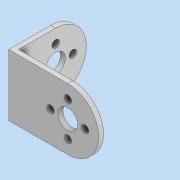
# Autodesk Inventor part: Bracket ANGULO
Saved by Autodesk Inventor 2021.4 (Build 254397000, 397)
## iProperties
Created: 2022-08-02
Part Number: Bracket ANGULO
Material: Generic
Document SubType Name: Modeling
Designer: ferbm
Density: 1 g/cm^3
Appearance: Default
Author: ferbm
Autodesk Inventor part; units mm, degrees
ref_plane "YZ Plane" through (0, 0, 0) normal (1, 0, 0) x (0, 1, 0)
ref_plane "XZ Plane" through (0, 0, 0) normal (0, 1, 0) x (-1, 0, 0)
ref_plane "XY Plane" through (0, 0, 0) normal (0, 0, 1) x (1, 0, 0)
sketch "Sketch1" plane through (0, 0, 0) normal (0, 0, 1) x (1, 0, 0)
  line L0 (0, 0) -> (24, 0)
  line L1 (24, 25) -> (0, 25)
  line L2 (0, 25) -> (0, 0)
  arc A0 (24, 0) -> (24, 25) centre (24, 12.5) ccw
  circle A1 centre (24, 12.5) radius 4
  circle A2 centre (24, 12.5) radius 7
  circle A3 centre (24, 19.5) radius 1.5
  circle A4 centre (17, 12.5) radius 1.5
  circle A5 centre (24, 5.5) radius 1.5
  circle A6 centre (31, 12.5) radius 1.5
  line L3 (24, 0) -> (24, 16.5)
  line L4 (24, 19.5) -> (24, 21)
  line L5 (0, 25) -> (2, 25)
  line L6 (2, 25) -> (2, 0)
  line L7 (2, 0) -> (0, 0)
  line L8 (0, 0) -> (0, 25)
  dimension "d2" = 8
  dimension "d3" = 14
  dimension "d4" = 3
  dimension "d0" = 24
  dimension "d1" = 25
  dimension "d7" = 360
  dimension "d11" = 2
  constraints: 18 end point, 5 parallel, 4 centre point, 3 perpendicular, 3 vertical alignment, 2 coincident, 2 horizontal, 2 point on circle, 2 tangent, 1 point on line, 15 other
  measures "d0" distance of L1.start L1.end
  measures "d1" distance of L0.end L1.start
  measures "d11" distance between parallel lines of L2 L6
extrude "Extrusion1" add sketch "Sketch1" along normal blind 2 contours L2 L1 L6 L0 | L6 L1 A0 L0 | A2 A4 A3 A6 A5
extrude "Extrusion2" add sketch "Sketch1" against normal blind 1 contours L2 L1 L6 L0
sketch "Sketch2" plane through (2, 0, 0) normal (1, 0, 0) x (0, 0, -1)
  line L0 (0, 25) -> (0, 0) projected
  line L1 (0, 25) -> (15, 25)
  line L2 (15, 25) -> (15, 0)
  line L3 (15, 0) -> (0, 0)
  line L4 (0, 0) -> (0, 25)
  circle A0 centre (15, 12.5) radius 12.5
  circle A1 centre (15, 12.5) radius 4
  circle A2 centre (15, 12.5) radius 7
  circle A3 centre (15, 19.5) radius 1.5
  circle A4 centre (8, 12.5) radius 1.5
  circle A5 centre (15, 5.5) radius 1.5
  circle A6 centre (22, 12.5) radius 1.5
  point P0 (15, 0)
  dimension "d17" = 14
  dimension "d14" = 15
  dimension "d15" = 25
  dimension "d16" = 8
  dimension "d18" = 3
  dimension "d21" = 360
  constraints: 8 end point, 6 centre point, 2 coincident, 2 parallel, 1 horizontal, 1 midpoint, 1 perpendicular, 1 point on line, 1 vertical alignment, 11 other
  measures "d14" distance of L2.end L3.end
  measures "d15" diameter of A0
  measures "d16" diameter of A1
  measures "d18" diameter of A3
extrude "Extrusion3" add sketch "Sketch2" against normal blind 2 contours L1 A0 L3 L0 | A0 L2 A5 A2 A6 A3 | L2 A3 A2 A4 A5 A0 | A3 L2 A1 A5 A2 A4 | A3 A2 A6 A5 L2 A1
body "Solid1"
